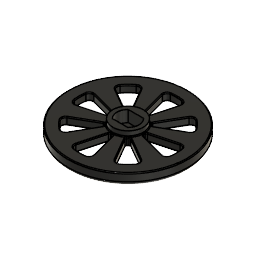
Wheel (Autodesk Fusion 360 design; units mm, degrees)
Autodesk Fusion 360 part; units mm, degrees
sketch "Wheel_Profile_Sketch" plane through (0, 0, 0) normal (0, 0, 1) x (1, 0, 0)
  line L0 (-3, 3) -> (3, -3) construction
  line L1 (3, 3) -> (-3, -3) construction
  arc A0 (3.0411, -3.1) -> (3.0411, 3.1) centre (0, 0) ccw
  line L2 (-3.0411, 3.1) -> (3.0411, 3.1)
  arc A1 (-3.0411, 3.1) -> (-3.0411, -3.1) centre (0, 0) ccw
  line L3 (3.0411, -3.1) -> (-3.0411, -3.1)
  circle A2 centre (0, 0) radius 6
  circle A3 centre (0, 0) radius 23.5
  line L4 (-4.2566, 5.4468) -> (-9.4968, 14.5231)
  line L5 (-5.3957, 4.3127) -> (-14.4768, 9.5557)
  line L6 (-1.0371, -18.9717) -> (-1.0371, -19)
  arc A4 (-4.3547, 4.8256) -> (-4.7781, 4.4067) centre (0, 0) ccw
  arc A5 (-11.7212, 14.9537) -> (-14.9034, 11.7851) centre (0, 0) ccw
  arc A6 (-14.9034, 11.7851) -> (-14.4768, 9.5557) centre (-13.7268, 10.8547) ccw
  arc A7 (-9.4968, 14.5231) -> (-11.7212, 14.9537) centre (-10.7959, 13.7731) ccw
  arc A8 (-5.3957, 4.3127) -> (-4.7781, 4.4067) centre (-5.1457, 4.7457) ccw
  arc A9 (-4.3547, 4.8256) -> (-4.2566, 5.4468) centre (-4.6896, 5.1968) ccw
  line L7 (-6.8649, -0.7658) -> (-16.9935, -3.4798)
  arc A10 (-18.862, 2.2857) -> (-18.8716, -2.2049) centre (0, 0) ccw
  arc A11 (-18.8716, -2.2049) -> (-16.9935, -3.4798) centre (-17.3818, -2.0309) ccw
  arc A12 (-16.9847, 3.5541) -> (-18.862, 2.2857) centre (-17.3729, 2.1052) ccw
  line L8 (-6.8614, 0.8416) -> (-16.9847, 3.5541)
  arc A13 (-6.8649, -0.7658) -> (-6.4947, -0.2626) centre (-6.9943, -0.2828) ccw
  arc A14 (-6.4915, 0.333) -> (-6.4947, -0.2626) centre (0, 0) ccw
  arc A15 (-6.4915, 0.333) -> (-6.8614, 0.8416) centre (-6.9908, 0.3586) ccw
  line L9 (-4.3127, -5.3957) -> (-9.5557, -14.4768)
  arc A16 (-14.9537, -11.7212) -> (-11.7851, -14.9034) centre (0, 0) ccw
  arc A17 (-11.7851, -14.9034) -> (-9.5557, -14.4768) centre (-10.8547, -13.7268) ccw
  arc A18 (-14.5231, -9.4968) -> (-14.9537, -11.7212) centre (-13.7731, -10.7959) ccw
  line L10 (-5.4468, -4.2566) -> (-14.5231, -9.4968)
  arc A19 (-4.3127, -5.3957) -> (-4.4067, -4.7781) centre (-4.7457, -5.1457) ccw
  arc A20 (-4.8256, -4.3547) -> (-4.4067, -4.7781) centre (0, 0) ccw
  arc A21 (-4.8256, -4.3547) -> (-5.4468, -4.2566) centre (-5.1968, -4.6896) ccw
  line L11 (0.7658, -6.8649) -> (3.4798, -16.9935)
  arc A22 (-2.2857, -18.862) -> (2.2049, -18.8716) centre (0, 0) ccw
  arc A23 (2.2049, -18.8716) -> (3.4798, -16.9935) centre (2.0309, -17.3818) ccw
  arc A24 (-3.5541, -16.9847) -> (-2.2857, -18.862) centre (-2.1052, -17.3729) ccw
  line L12 (-0.8416, -6.8614) -> (-3.5541, -16.9847)
  arc A25 (0.7658, -6.8649) -> (0.2626, -6.4947) centre (0.2828, -6.9943) ccw
  arc A26 (-0.333, -6.4915) -> (0.2626, -6.4947) centre (0, 0) ccw
  arc A27 (-0.333, -6.4915) -> (-0.8416, -6.8614) centre (-0.3586, -6.9908) ccw
  line L13 (5.3957, -4.3127) -> (14.4768, -9.5557)
  arc A28 (11.7212, -14.9537) -> (14.9034, -11.7851) centre (0, 0) ccw
  arc A29 (14.9034, -11.7851) -> (14.4768, -9.5557) centre (13.7268, -10.8547) ccw
  arc A30 (9.4968, -14.5231) -> (11.7212, -14.9537) centre (10.7959, -13.7731) ccw
  line L14 (4.2566, -5.4468) -> (9.4968, -14.5231)
  arc A31 (5.3957, -4.3127) -> (4.7781, -4.4067) centre (5.1457, -4.7457) ccw
  arc A32 (4.3547, -4.8256) -> (4.7781, -4.4067) centre (0, 0) ccw
  arc A33 (4.3547, -4.8256) -> (4.2566, -5.4468) centre (4.6896, -5.1968) ccw
  line L15 (6.8649, 0.7658) -> (16.9935, 3.4798)
  arc A34 (18.862, -2.2857) -> (18.8716, 2.2049) centre (0, 0) ccw
  arc A35 (18.8716, 2.2049) -> (16.9935, 3.4798) centre (17.3818, 2.0309) ccw
  arc A36 (16.9847, -3.5541) -> (18.862, -2.2857) centre (17.3729, -2.1052) ccw
  line L16 (6.8614, -0.8416) -> (16.9847, -3.5541)
  arc A37 (6.8649, 0.7658) -> (6.4947, 0.2626) centre (6.9943, 0.2828) ccw
  arc A38 (6.4915, -0.333) -> (6.4947, 0.2626) centre (0, 0) ccw
  arc A39 (6.4915, -0.333) -> (6.8614, -0.8416) centre (6.9908, -0.3586) ccw
  line L17 (4.3127, 5.3957) -> (9.5557, 14.4768)
  arc A40 (14.9537, 11.7212) -> (11.7851, 14.9034) centre (0, 0) ccw
  arc A41 (11.7851, 14.9034) -> (9.5557, 14.4768) centre (10.8547, 13.7268) ccw
  arc A42 (14.5231, 9.4968) -> (14.9537, 11.7212) centre (13.7731, 10.7959) ccw
  line L18 (5.4468, 4.2566) -> (14.5231, 9.4968)
  arc A43 (4.3127, 5.3957) -> (4.4067, 4.7781) centre (4.7457, 5.1457) ccw
  arc A44 (4.8256, 4.3547) -> (4.4067, 4.7781) centre (0, 0) ccw
  arc A45 (4.8256, 4.3547) -> (5.4468, 4.2566) centre (5.1968, 4.6896) ccw
  line L19 (-0.7658, 6.8649) -> (-3.4798, 16.9935)
  arc A46 (2.2857, 18.862) -> (-2.2049, 18.8716) centre (0, 0) ccw
  arc A47 (-2.2049, 18.8716) -> (-3.4798, 16.9935) centre (-2.0309, 17.3818) ccw
  arc A48 (3.5541, 16.9847) -> (2.2857, 18.862) centre (2.1052, 17.3729) ccw
  line L20 (0.8416, 6.8614) -> (3.5541, 16.9847)
  arc A49 (-0.7658, 6.8649) -> (-0.2626, 6.4947) centre (-0.2828, 6.9943) ccw
  arc A50 (0.333, 6.4915) -> (-0.2626, 6.4947) centre (0, 0) ccw
  arc A51 (0.333, 6.4915) -> (0.8416, 6.8614) centre (0.3586, 6.9908) ccw
  dimension "d1" = 6
  dimension "d2" = 6
  dimension "d4" = 12
  dimension "d5" = 6.2
  dimension "d6" = 47
  dimension "d13" = 1.5
  dimension "d14" = 1.5
  dimension "d15" = 0.5
  dimension "d16" = 0.5
  dimension "d18" = 360
  constraint midpoint A0.centre L1
  constraint concentric A1 A3
  constraint tangent A5 A6
  constraint tangent L5 A6
  constraint tangent A5 A7
  constraint tangent L4 A7
  constraint tangent L5 A8
  constraint tangent A4 A8
  constraint tangent L4 A9
  constraint tangent A4 A9
  measures "d1" distance of L0.start L1.start
  measures "d2" distance of L0.start L1.end
  measures "d4" diameter of A2
  measures "d5" distance of L2.start A1.end
  measures "d6" diameter of A3
  measures "d13" radius of A6
  measures "d14" radius of A7
  measures "d15" radius of A8
  measures "d16" radius of A9
extrude "Extrude1" add sketch "Wheel_Profile_Sketch" along normal blind 3 contours A0 L2 A1 L3 | A2 | A3
extrude "Extrude2" add sketch "Wheel_Profile_Sketch" along normal blind 5 contours A2
extrude "Extrude3" cut sketch "Wheel_Profile_Sketch" along normal blind 5 from surface at 0.5 contours A0 L2 A1 L3
torus "TorusPrimitive1" add centre line diameter 44 section diameter 3 placed x (1, 0, 0) y (0, -1, 0) z (0, 0, -1) at (0, 0, 0)
fillet "Fillet1" radius 0.4 1 faces at (-12.3212, -5.7444, 0)
fillet "Fillet2" radius 0.3 1 faces at (-12.3212, -5.7444, 3)
named bodies: "Drive_Wheel_Body"
